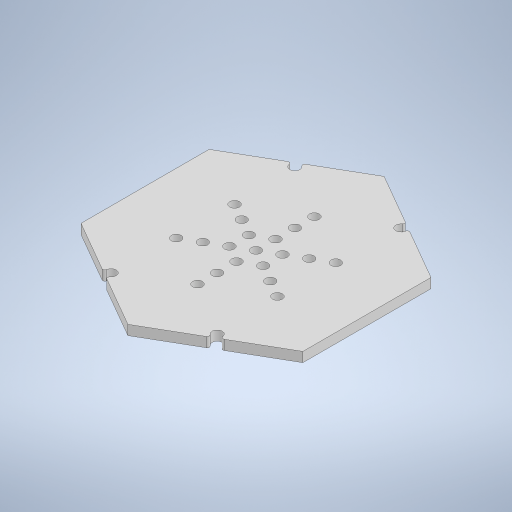
# Autodesk Inventor part: top
Saved by Autodesk Inventor 2024 (Build 280153000, 153)
## iProperties
Created: 2024-03-18
Part Number: top
Material: 일반
Document SubType Name: Modeling
Designer: SSAFY
Density: 1 g/cm^3
Appearance: 기본값
Author: SSAFY
Autodesk Inventor part; units mm, degrees
ref_plane "YZ Plane" through (0, 0, 0) normal (1, 0, 0) x (0, 1, 0)
ref_plane "XZ Plane" through (0, 0, 0) normal (0, 1, 0) x (-1, 0, 0)
ref_plane "XY Plane" through (0, 0, 0) normal (0, 0, 1) x (1, 0, 0)
sketch "스케치2" plane through (0, 0, 0) normal (0, 1, 0) x (-1, 0, 0)
  line L0 (0, 60) -> (51.9615, 30)
  line L1 (51.9615, 30) -> (51.9615, -30)
  line L2 (51.9615, -30) -> (0, -60)
  line L3 (0, -60) -> (-51.9615, -30)
  line L4 (-51.9615, -30) -> (-51.9615, 30)
  line L5 (-51.9615, 30) -> (0, 60)
  line L6 (0, 65.7735) -> (56.9615, 32.8868)
  line L7 (56.9615, 32.8868) -> (56.9615, -32.8868)
  line L8 (56.9615, -32.8868) -> (0, -65.7735)
  line L9 (0, -65.7735) -> (-56.9615, -32.8868)
  line L10 (-56.9615, -32.8868) -> (-56.9615, 32.8868)
  line L11 (-56.9615, 32.8868) -> (0, 65.7735)
  circle A0 centre (-54.4615, 0) radius 2.5 construction
  circle A1 centre (-54.4615, 0) radius 2.6
  circle A2 centre (-27.2308, -47.1651) radius 2.5 construction
  circle A3 centre (-27.2308, -47.1651) radius 2.6
  circle A4 centre (27.2308, -47.1651) radius 2.5 construction
  circle A5 centre (27.2308, -47.1651) radius 2.6
  circle A6 centre (54.4615, 0) radius 2.5 construction
  circle A7 centre (54.4615, 0) radius 2.6
  circle A8 centre (27.2308, 47.1651) radius 2.5 construction
  circle A9 centre (27.2308, 47.1651) radius 2.6
  circle A10 centre (-27.2308, 47.1651) radius 2.5 construction
  circle A11 centre (-27.2308, 47.1651) radius 2.6
  point P0 (0, 0)
  point P1 (0, 0)
  point P2 (-56.9615, -0.7141)
  point P3 (-29.0992, -48.9731)
  point P4 (-27.8623, -49.6872)
  point P5 (27.8623, -49.6872)
  point P6 (29.0992, -48.9731)
  point P7 (56.9615, -0.7141)
  point P8 (56.9615, 0.7141)
  point P9 (29.0992, 48.9731)
  point P10 (27.8623, 49.6872)
  point P11 (-27.8623, 49.6872)
  point P12 (-29.0992, 48.9731)
  point P13 (-56.9615, 0.7141)
  point P14 (25.3623, -45.3571)
  point P15 (26.5992, -44.6429)
  dimension "d0" = 60
  dimension "d1" = 5
  dimension "d2" = 5
  dimension "d3" = 5.2
  dimension "d6" = 360
  constraints: 24 end point, 12 centre point, 7 coincident, 1 tangent, 43 other
  measures "d0" distance of L3.end L4.end
  measures "d1" distance between parallel lines of L10 L4
  measures "d2" diameter of A0
  measures "d3" diameter of A1
extrude "돌출1" add sketch "스케치2" along normal blind 5 contours L5 A11 L11 L6 A9 L0 | L0 A9 L1 A7 L2 A5 L3 A3 L4 A1 L5 A11 | A9 L6 L7 A7 L1 L0 | L5 L4 A1 L10 L11 A11 | A7 L7 L1 | L1 A7 | A1 L4 | L4 A1 L10 | A7 L7 L8 A5 L2 L1 | L4 L3 A3 L9 L10 A1 | L2 A5 | A5 L8 L9 A3 L3 L2
fillet "모깎기1" radius 1 8 edges at (-29.0992, 2.5, 48.9731) (-27.8623, 2.5, 49.6872) (27.8623, 2.5, 49.6872) (29.0992, 2.5, 48.9731) (27.8623, 2.5, -49.6872) (29.0992, 2.5, -48.9731) (-29.0992, 2.5, -48.9731) (-27.8623, 2.5, -49.6872)
sketch "스케치3" plane through (0, 5, 0) normal (0, 1, 0) x (1, 0, 0)
  circle A0 centre (0, 0) radius 2.5
  line L0 (0, 10) -> (8.6603, 5)
  line L1 (8.6603, 5) -> (8.6603, -5)
  line L2 (8.6603, -5) -> (0, -10)
  line L3 (0, -10) -> (-8.6603, -5)
  line L4 (-8.6603, -5) -> (-8.6603, 5)
  line L5 (-8.6603, 5) -> (0, 10)
  line L6 (0, 20) -> (17.3205, 10)
  line L7 (17.3205, 10) -> (17.3205, -10)
  line L8 (17.3205, -10) -> (0, -20)
  line L9 (0, -20) -> (-17.3205, -10)
  line L10 (-17.3205, -10) -> (-17.3205, 10)
  line L11 (-17.3205, 10) -> (0, 20)
  line L12 (0, 30) -> (25.9808, 15)
  line L13 (25.9808, 15) -> (25.9808, -15)
  line L14 (25.9808, -15) -> (0, -30)
  line L15 (0, -30) -> (-25.9808, -15)
  line L16 (-25.9808, -15) -> (-25.9808, 15)
  line L17 (-25.9808, 15) -> (0, 30)
  circle A1 centre (0, 10) radius 2.5
  circle A2 centre (0, 20) radius 2.5
  circle A3 centre (0, 30) radius 2.5
  circle A4 centre (-25.9808, 15) radius 2.5
  circle A5 centre (-17.3205, 10) radius 2.5
  circle A6 centre (-8.6603, 5) radius 2.5
  circle A7 centre (-25.9808, -15) radius 2.5
  circle A8 centre (-17.3205, -10) radius 2.5
  circle A9 centre (-8.6603, -5) radius 2.5
  circle A10 centre (0, -30) radius 2.5
  circle A11 centre (0, -20) radius 2.5
  circle A12 centre (0, -10) radius 2.5
  circle A13 centre (25.9808, -15) radius 2.5
  circle A14 centre (17.3205, -10) radius 2.5
  circle A15 centre (8.6603, -5) radius 2.5
  circle A16 centre (25.9808, 15) radius 2.5
  circle A17 centre (17.3205, 10) radius 2.5
  circle A18 centre (8.6603, 5) radius 2.5
  dimension "d11" = 5
  dimension "d12" = 10
  dimension "d13" = 20
  dimension "d14" = 30
  dimension "d17" = 360
  constraints: 36 end point, 19 centre point, 7 coincident, 76 other
  measures "d11" diameter of A0
  measures "d12" distance of L3.end L4.end
  measures "d13" distance of L9.end L10.end
  measures "d14" distance of L15.end L16.end
extrude "돌출2" cut sketch "스케치3" against normal through all contours A0 | L5 A1 L0 | L0 A1 L5 | A18 L1 L0 | L0 L1 A18 | A6 L4 L5 | L5 L4 A6 | A15 L2 L1 | L1 L2 A15 | A9 L3 L4 | L4 L3 A9 | A12 L3 L2 | L2 L3 A12 | L11 A2 L6 | L6 A2 L11 | A17 L7 L6 | L6 L7 A17 | A5 L10 L11 | L11 L10 A5 | A14 L8 L7 | L7 L8 A14 | A8 L9 L10 | L10 L9 A8 | A11 L9 L8 | L8 L9 A11 | L17 A3 L12 | L12 A3 L17 | A16 L13 L12 | L12 L13 A16 | A4 L16 L17 | L17 L16 A4 | A13 L14 L13 | L13 L14 A13 | A7 L15 L16 | L16 L15 A7 | A10 L15 L14 | L14 L15 A10
